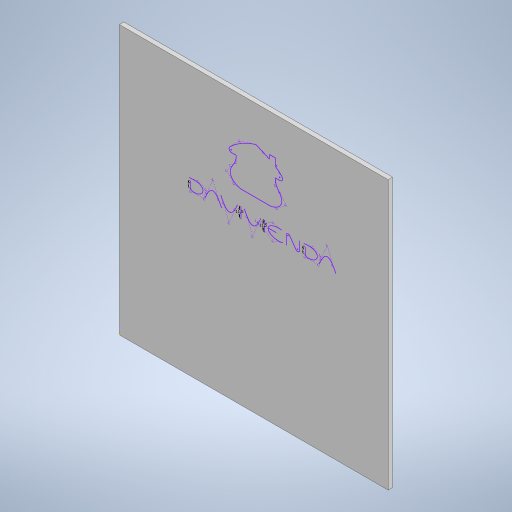
# Autodesk Inventor part: Davivienda
Saved by Autodesk Inventor 2023 (Build 270158000, 158)
## iProperties
Created: 2024-11-21
Part Number: Davivienda
Material: Generic
Document SubType Name: Modeling
Designer: Zenbook
Density: 1 g/cm^3
Appearance: Default
Author: Zenbook
Autodesk Inventor part; units mm, degrees
ref_plane "YZ Plane" through (0, 0, 0) normal (1, 0, 0) x (0, 1, 0)
ref_plane "XZ Plane" through (0, 0, 0) normal (0, 1, 0) x (-1, 0, 0)
ref_plane "XY Plane" through (0, 0, 0) normal (0, 0, 1) x (1, 0, 0)
sketch "Sketch2" plane through (0, 0, 0) normal (0, 0, 1) x (1, 0, 0)
  line L0 (0, 0) -> (300, 0)
  line L1 (300, 0) -> (300, 300)
  line L2 (300, 300) -> (0, 300)
  line L3 (0, 300) -> (0, 0)
  dimension "d0" = 300
  dimension "d1" = 300
  constraints: 8 end point, 2 parallel, 1 horizontal, 1 perpendicular
  measures "d0" distance of L2.end L1.end
  measures "d1" distance of L1.end L0.end
extrude "Extrusion1" add sketch "Sketch2" along normal blind 5
sketch "Sketch4" plane through (0, 0, 5) normal (0, 0, 1) x (1, 0, 0)
  line L0 (79.5564, 188.2855) -> (79.5564, 181.2855)
  line L1 (79.5564, 181.2855) -> (79.5564, 178.6599) construction
  line L2 (79.5564, 178.6599) -> (94.7024, 178.6599) construction
  line L3 (94.7024, 178.6599) -> (96.5971, 188.6652) construction
  line L4 (96.5971, 188.6652) -> (88.3362, 192.4913) construction
  line L5 (88.3362, 192.4913) -> (77.7258, 191.1271) construction
  spline S0 degree 4 poles (79.5564, 181.2855) (79.5564, 178.6599) (94.7024, 178.6599) (96.5971, 188.6652) (88.3362, 192.4913) (77.7258, 191.1271) knots 1 1 1 1 1 2 3 3 3 3 3
  line L6 (95.2867, 179.9727) -> (97.8294, 186.2811) construction
  line L7 (97.8294, 186.2811) -> (104.3309, 202.3418) construction
  line L8 (104.3309, 202.3418) -> (110.5428, 186.2811) construction
  line L9 (110.5428, 186.2811) -> (113.8579, 179.9727) construction
  spline S1 degree 4 poles (95.2867, 179.9727) (97.8294, 186.2811) (104.3309, 202.3418) (110.5428, 186.2811) (113.8579, 179.9727) knots 1 1 1 1 1 2 2 2 2 2
  line L10 (131.5825, 191.7075) -> (129.0398, 185.3991) construction
  line L11 (129.0398, 185.3991) -> (122.5383, 169.3383) construction
  line L12 (122.5383, 169.3383) -> (116.3264, 185.3991) construction
  line L13 (116.3264, 185.3991) -> (113.0113, 191.7075) construction
  spline S2 degree 4 poles (131.5825, 191.7075) (129.0398, 185.3991) (122.5383, 169.3383) (116.3264, 185.3991) (113.0113, 191.7075) knots 1 1 1 1 1 2 2 2 2 2
  spline S3 degree 4 poles (157.762, 191.8087) (155.2194, 185.5002) (148.7178, 169.4395) (142.5059, 185.5002) (139.1908, 191.8087) knots 1 1 1 1 1 2 2 2 2 2
  line L14 (157.762, 191.8087) -> (155.2194, 185.5002) construction
  line L15 (155.2194, 185.5002) -> (148.7178, 169.4395) construction
  line L16 (148.7178, 169.4395) -> (142.5059, 185.5002) construction
  line L17 (142.5059, 185.5002) -> (139.1908, 191.8087) construction
  line L18 (135.5149, 191.7075) -> (135.5149, 180.2075)
  line L19 (162.0018, 191.8085) -> (162.0018, 180.3085)
  line L20 (180.6346, 191.8085) -> (171.5415, 194.3115) construction
  line L21 (171.5415, 194.3115) -> (152.9228, 186.4259) construction
  line L22 (152.9228, 186.4259) -> (171.5415, 176.543) construction
  line L23 (171.5415, 176.543) -> (182.4118, 180.3085) construction
  spline S4 degree 4 poles (180.6346, 191.8085) (171.5415, 194.3115) (152.9228, 186.4259) (171.5415, 176.543) (182.4118, 180.3085) knots 1 1 1 1 1 2 2 2 2 2
  line L24 (165.8328, 186.4259) -> (174.8813, 186.4259)
  line L25 (186.057, 180.0241) -> (186.057, 189.935)
  line L26 (189.8603, 191.1584) -> (197.0204, 180.9967)
  line L27 (201.0713, 182.1524) -> (201.0713, 191.8085)
  arc A0 (189.8811, 191.1289) -> (186.057, 189.935) centre (188.1554, 189.935) ccw
  arc A1 (197.0204, 180.9967) -> (201.0713, 182.1524) centre (198.8441, 182.2817) ccw
  line L28 (207.2296, 188.507) -> (207.2296, 181.507)
  line L29 (207.2296, 181.507) -> (207.2296, 178.8814) construction
  line L30 (207.2296, 178.8814) -> (222.3756, 178.8814) construction
  line L31 (222.3756, 178.8814) -> (224.2703, 188.8868) construction
  line L32 (224.2703, 188.8868) -> (216.0093, 192.7129) construction
  line L33 (216.0093, 192.7129) -> (205.3989, 191.3487) construction
  spline S5 degree 4 poles (207.2296, 181.507) (207.2296, 178.8814) (222.3756, 178.8814) (224.2703, 188.8868) (216.0093, 192.7129) (205.3989, 191.3487) knots 1 1 1 1 1 2 3 3 3 3 3
  line L34 (222.9422, 180.0767) -> (225.4849, 186.3851) construction
  line L35 (225.4849, 186.3851) -> (231.9865, 202.4459) construction
  line L36 (231.9865, 202.4459) -> (238.1983, 186.3851) construction
  line L37 (238.1983, 186.3851) -> (241.5135, 180.0767) construction
  spline S6 degree 4 poles (222.9422, 180.0767) (225.4849, 186.3851) (231.9865, 202.4459) (238.1983, 186.3851) (241.5135, 180.0767) knots 1 1 1 1 1 2 2 2 2 2
  line L38 (135.9918, 208.9074) -> (168.4766, 208.9074)
  line L39 (167.2414, 253.646) -> (167.2414, 258.1826)
  line L40 (167.2414, 258.1826) -> (173.7908, 258.1826)
  line L41 (173.7908, 258.1826) -> (173.7908, 249.9244)
  line L42 (135.9918, 208.9074) -> (128.025, 210.0808) construction
  line L43 (128.025, 210.0808) -> (119.7557, 218.4745) construction
  line L44 (119.7557, 218.4745) -> (124.3195, 226.1379) construction
  line L45 (124.3195, 226.1379) -> (130.2483, 231.5726) construction
  line L46 (130.2483, 231.5726) -> (130.2483, 238.8487) construction
  spline S7 degree 4 poles (135.9918, 208.9074) (128.025, 210.0808) (119.7557, 218.4745) (124.3195, 226.1379) (130.2483, 231.5726) (130.2483, 238.8487) knots 1 1 1 1 1 2 3 3 3 3 3
  line L47 (168.4766, 208.9074) -> (175.8602, 210.0808) construction
  line L48 (175.8602, 210.0808) -> (186.1394, 218.4745) construction
  line L49 (186.1394, 218.4745) -> (179.0921, 227.5218) construction
  line L50 (179.0921, 227.5218) -> (173.9355, 231.5726) construction
  line L51 (173.9355, 231.5726) -> (173.9355, 238.8487) construction
  spline S8 degree 4 poles (168.4766, 208.9074) (175.8602, 210.0808) (186.1394, 218.4745) (179.0921, 227.5218) (173.9355, 231.5726) (173.9355, 238.8487) knots 1 1 1 1 1 2 3 3 3 3 3
  line L52 (123.2696, 243.6155) -> (134.5896, 254.6512) construction
  line L53 (134.5896, 254.6512) -> (152.0248, 260.2524) construction
  spline S9 degree 2 poles (123.2696, 243.6155) (134.5896, 254.6512) (152.0248, 260.2524) knots 1 1 1 2 2 2
  line L54 (152.0248, 260.2524) -> (160.8389, 256.9124) construction
  line L55 (179.2014, 246.4492) -> (181.8101, 243.0596) construction
  arc A2 (123.2696, 243.6155) -> (124.9575, 238.8487) centre (124.9575, 241.5309) ccw
  arc A3 (179.0921, 238.8487) -> (181.8101, 243.0596) centre (179.0921, 241.8313) ccw
  line L56 (124.9575, 238.8487) -> (130.2483, 238.8487)
  line L57 (173.9355, 238.8487) -> (179.0921, 238.8487)
  spline S10 degree 2 poles (152.0248, 260.2524) (160.8389, 256.9124) (167.2414, 253.646) knots 0 0 0 1 1 1
  spline S11 degree 2 poles (173.7908, 249.9244) (179.2014, 246.4492) (181.8101, 243.0596) knots 0 0 0 1 1 1
  line L58 (160.8389, 256.9124) -> (167.2414, 253.646) construction
  line L59 (173.7908, 249.9244) -> (179.2014, 246.4492) construction
  point P0 (0, 0)
  point P1 (175.3935, 251.397)
  dimension "d11" = 7
  dimension "d28" = 11.5
  dimension "d29" = 11.5
  dimension "d42" = 7
  constraints: 28 end point, 9 point on circle, 7 vertical, 6 tangent, 4 centre point, 4 horizontal, 4 perpendicular, 1 point on line, 37 other
  measures "d11" distance of L0.start L0.end
  measures "d28" distance of L18.start L18.end
  measures "d29" distance of L19.start L19.end
  measures "d42" distance of L28.start L29.start
body "Solid1"
